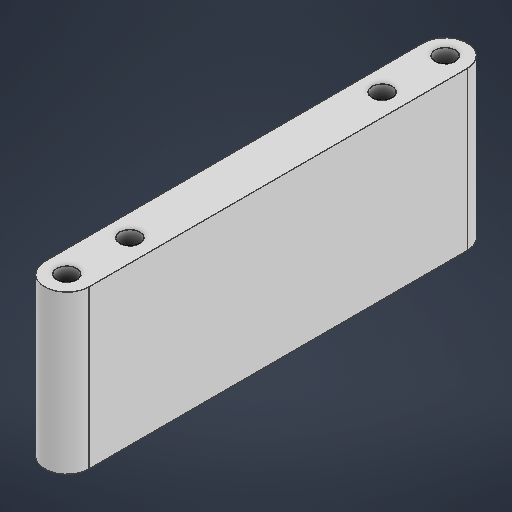
# Autodesk Inventor part: cover_wall_1
Saved by Autodesk Inventor 2026.1 (Build 301233000, 233)
## iProperties
Created: 2026-03-31
Part Number: cover_wall_1
Material: Generic
Document SubType Name: Modeling
Designer: emanuel
Density: 1 g/cm^3
Appearance: Default
Author: emanuel
Autodesk Inventor part; units mm, degrees
ref_plane "YZ Plane" through (0, 0, 0) normal (1, 0, 0) x (0, 1, 0)
ref_plane "XZ Plane" through (0, 0, 0) normal (0, 1, 0) x (-1, 0, 0)
ref_plane "XY Plane" through (0, 0, 0) normal (0, 0, 1) x (1, 0, 0)
sketch "Sketch1" plane through (0, 0, 0) normal (0, 1, 0) x (-1, 0, 0)
  circle A0 centre (0, 0) radius 1.6
  line L0 (0, 0) -> (0, -10)
  circle A1 centre (0, -10) radius 1.6
  line L1 (0, 0) -> (0, 40)
  circle A2 centre (0, 40) radius 1.6
  line L2 (0, 40) -> (0, 50)
  circle A3 centre (0, 50) radius 1.6
  line L3 (0, 50) -> (0, -10) construction
  line L4 (-3.5, 50) -> (-3.5, -10)
  line L5 (3.5, -10) -> (3.5, 50)
  arc A4 (3.5, 50) -> (-3.5, 50) centre (0, 50) ccw
  arc A5 (-3.5, -10) -> (3.5, -10) centre (0, -10) ccw
  point P0 (0, 20)
  dimension "d0" = 3.2
  dimension "d1" = 10
  dimension "d2" = 3.2
  dimension "d3" = 40
  dimension "d4" = 3.2
  dimension "d5" = 10
  dimension "d6" = 3.2
  dimension "d7" = 7
  constraints: 14 end point, 6 centre point, 4 coincident, 4 point on circle, 4 tangent, 4 vertical, 1 midpoint, 1 parallel
  measures "d0" diameter of A0
  measures "d1" distance of L0.start L0.end
  measures "d2" diameter of A1
  measures "d3" distance of L0.start L1.end
  measures "d4" diameter of A2
  measures "d5" distance of L2.start L2.end
  measures "d6" diameter of A3
  measures "d7" diameter of A5
extrude "Extrusion1" add sketch "Sketch1" along normal blind 25
body "Solid1"
